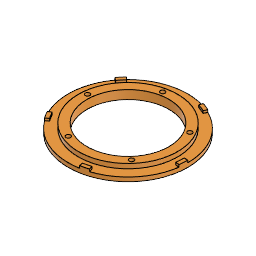
Frame-Top (Autodesk Fusion 360 design; units mm, degrees)
part number: 2026-05-19-19-00-25-859
Autodesk Fusion 360 part; units mm, degrees
sketch "Sketch1" plane through (0, 0, 0) normal (0, 0, 1) x (1, 0, 0)
  circle A0 centre (0, 0) radius 65
  circle A1 centre (0, 0) radius 44.5
  circle A2 centre (0, 0) radius 54
  line L0 (44.5, 30.59) -> (44.5, 0) construction
  line L1 (-10.3681, 43.2753) -> (-10.3681, 52.9953) construction
  circle A3 centre (-10.3681, 48.1353) radius 2.5
  circle A4 centre (-48.9833, 5.014) radius 2.5
  circle A5 centre (-19.9052, -45.0365) radius 2.5
  circle A6 centre (36.6812, -32.8481) radius 2.5
  circle A7 centre (42.5755, 24.7353) radius 2.5
  line L2 (0, 0) -> (65, 0) construction
  line L3 (0, 0) -> (65, 0) construction
  line L4 (18.85, 58.0144) -> (20.0861, 61.8187)
  line L5 (26.7406, 54.8264) -> (28.4941, 58.4216)
  line L6 (-49.35, 35.8549) -> (-52.5861, 38.206)
  line L7 (-43.8797, 42.3742) -> (-46.7571, 45.1528)
  line L8 (-49.35, -35.8549) -> (-52.5861, -38.206)
  line L9 (-53.8598, -28.6378) -> (-57.3916, -30.5157)
  line L10 (18.85, -58.0144) -> (20.0861, -61.8187)
  line L11 (10.5925, -60.0733) -> (11.2871, -64.0125)
  line L12 (61, 0) -> (65, 0)
  line L13 (60.4064, -8.4896) -> (64.3674, -9.0463)
  arc A8 (26.7406, 54.8264) -> (18.85, 58.0144) centre (0, 0) ccw
  arc A9 (60.4064, -8.4896) -> (61, 0) centre (0, 0) ccw
  arc A10 (-43.8797, 42.3742) -> (-49.35, 35.8549) centre (0, 0) ccw
  arc A11 (-53.8598, -28.6378) -> (-49.35, -35.8549) centre (0, 0) ccw
  arc A12 (10.5925, -60.0733) -> (18.85, -58.0144) centre (0, 0) ccw
  line L14 (0, 0) -> (42.5755, 24.7353) construction
  line L15 (0, 0) -> (0, -65) construction
  dimension "d1" = 130
  dimension "d2" = 89
  dimension "d3" = 108
  dimension "d4" = 5
  dimension "d6" = 360
  dimension "d11" = 360
  dimension "d22" = 30.156
  dimension "d23" = 61
  dimension "d24" = 10
  dimension "d26" = 18
  constraint coincident A0.centre A1.centre
  constraint concentric A1 A2
  constraint coincident A2 L0.start
  constraint coincident A1 L0.end
  constraint vertical L0
  constraint tangent A1 L0
  constraint coincident A2 L1.end
  constraint vertical L1
  constraint coincident A1 L1.start
  constraint midpoint L1 A3.centre
  constraint horizontal L2
  constraint coincident A0 L5.end
  constraint horizontal L3
  constraint coincident A0 L4.end
  constraint concentric A0 A10
  constraint concentric A8 A9
  constraint concentric A9 A12
  constraint concentric A10 A11
  constraint concentric A11 A12
  constraint coincident A7.centre L14.end
  constraint coincident L11 A0.centre
  constraint coincident A0.centre L10
  constraint coincident A0 L15.end
  constraint vertical L15
  measures "d1" diameter of A0
  measures "d2" diameter of A1
  measures "d3" diameter of A2
  measures "d4" diameter of A3
  measures "d22" angle of L2 L14
  measures "d23" radius of A12
  measures "d24" angle of L11 L15
  measures "d26" angle of L10 L15
extrude "Extrude1" add sketch "Sketch1" along normal blind 7 contours A0 L12 L13 A9 | A0 L4 L5 A8 | A0 L10 L11 A12 | A0 L6 L7 A10 | A0 L8 L9 A11 makes body 1 at (64.8749, -4.0311, 4.6667) makes body 2 at (21.9942, 61.1658, 4.6667) makes body 3 at (16.2137, -62.9453, 4.6667) makes body 4 at (-51.9871, 39.0172, 4.6667) makes body 5 at (-53.1725, -37.3857, 4.6667)
extrude "Extrude2" add sketch "Sketch1" along normal blind 4.5 contours A0 L4 L5 L6 L7 L8 L9 L10 L11 L12 L13 A8 A9 A10 A11 A12 bodies 1 2 3 4 5
extrude "Extrude3" add sketch "Sketch1" along normal blind 9.5 contours A2 bodies 1
extrude "Extrude4" add sketch "Sketch1" along normal blind 1.5 contours A3 | A4 | A5 | A6 | A7 bodies 1
